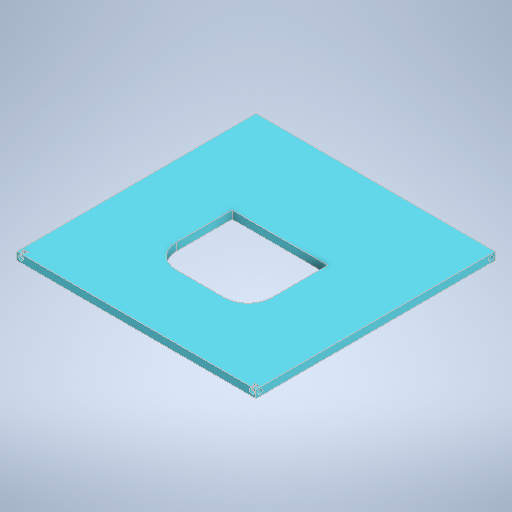
# Autodesk Inventor part: CasaJugueteAPM
Saved by Autodesk Inventor 2025.2 (Build 292293000, 293)
## iProperties
Created: 2024-11-26
Part Number: CasaJugueteAPM
Material: Plástico ABS
Document SubType Name: Modeling
Designer: usuario
Density: 1.06 g/cm^3
Appearance: Suave - Negro
Author: usuario
Autodesk Inventor part; units mm, degrees
ref_plane "YZ Plane" through (0, 0, 0) normal (1, 0, 0) x (0, 1, 0)
ref_plane "XZ Plane" through (0, 0, 0) normal (0, 1, 0) x (-1, 0, 0)
ref_plane "XY Plane" through (0, 0, 0) normal (0, 0, 1) x (1, 0, 0)
sketch "Boceto1" plane through (0, 0, 0) normal (0, 0, 1) x (1, 0, 0)
  line L0 (0, 0) -> (150, 0)
  line L1 (150, 0) -> (150, 150)
  line L2 (150, 150) -> (0, 150)
  line L3 (0, 150) -> (0, 0)
  line L4 (5, 145) -> (145, 145)
  line L5 (145, 145) -> (145, 5)
  line L6 (145, 5) -> (5, 5)
  line L7 (5, 5) -> (5, 145)
  dimension "d0" = 150
  dimension "d1" = 150
  dimension "d2" = 5
  constraints: 16 end point, 4 parallel, 2 perpendicular, 1 horizontal, 3 other
  measures "d0" distance of L2.end L1.end
  measures "d1" distance of L1.end L0.end
  measures "d2" distance between parallel lines of L2 L4
extrude "Extrusión1" add sketch "Boceto1" along normal blind 150
sketch "Boceto2" plane through (150, 0, 0) normal (1, 0, 0) x (0, 0, -1)
  line L0 (-150, 0) -> (-150, 150) projected
  line L1 (-150, 75) -> (-190, 75) construction
  line L2 (-190, 75) -> (-150, 150)
  line L3 (0, 0) -> (-150, 0) construction
  line L4 (-150, 0) -> (-190, 75)
  dimension "d5" = 40
  constraints: 6 end point, 1 horizontal, 1 midpoint
  measures "d5" distance of L1.start L1.end
extrude "Extrusión2" add sketch "Boceto2" against normal blind 5
ref_plane "Plano de trabajo1" through (75, 0, 0) normal (1, 0, 0) x (0, 0, -1)
mirror "Simetría1" about plane through (75, 0, 0) normal (1, 0, 0) of "Extrusión2"
sketch "Boceto3" plane through (0, 150, 0) normal (0, 1, 0) x (1, 0, 0)
  line L0 (105, -60) -> (45, -60)
  line L1 (45, -60) -> (45, -95)
  line L2 (60, -110) -> (90, -110)
  line L3 (105, -95) -> (105, -60)
  line L4 (150, 0) -> (0, 0) projected
  line L5 (145, -150) -> (5, -150) projected
  arc A0 (90, -110) -> (105, -95) centre (90, -95) ccw
  arc A1 (45, -95) -> (60, -110) centre (60, -95) ccw
  point P0 (45, -110)
  point P1 (105, -110)
  point P2 (75, -60)
  point P3 (75, 0)
  dimension "d8" = 60
  dimension "d9" = 50
  dimension "d10" = 40
  dimension "d11" = 15
  constraints: 8 end point, 4 point on circle, 4 point on line, 4 tangent, 2 centre point, 2 midpoint, 2 parallel, 1 equal radius, 1 horizontal, 1 perpendicular, 1 vertical alignment
  measures "d8" distance of point (105, -110) point (45, -110)
  measures "d9" distance of point (45, -110) L0.end
  measures "d10" distance between parallel lines of L5 L2
  measures "d11" radius of A0
extrude "Extrusión3" cut sketch "Boceto3" against normal through all
sketch "Boceto4" plane through (150, 0, 0) normal (1, 0, 0) x (0, 0, -1)
  line L0 (-13, 20) -> (-123, 20)
  line L1 (-128, 25) -> (-128, 75)
  line L2 (-123, 80) -> (-13, 80)
  line L3 (-8, 75) -> (-8, 25)
  line L4 (0, 0) -> (0, 150) projected
  line L5 (0, 0) -> (-150, 0) projected
  arc A0 (-123, 80) -> (-128, 75) centre (-123, 75) ccw
  arc A1 (-8, 75) -> (-13, 80) centre (-13, 75) ccw
  arc A2 (-13, 20) -> (-8, 25) centre (-13, 25) ccw
  arc A3 (-128, 25) -> (-123, 20) centre (-123, 25) ccw
  point P0 (-128, 80)
  point P1 (-128, 20)
  point P2 (-8, 80)
  dimension "d14" = 120
  dimension "d15" = 60
  dimension "d16" = 8
  dimension "d17" = 20
  dimension "d18" = 5
  constraints: 8 end point, 8 point on circle, 8 tangent, 6 point on line, 4 centre point, 3 equal radius, 2 parallel, 1 horizontal, 1 perpendicular
  measures "d14" distance of point (-128, 80) point (-8, 80)
  measures "d15" distance of point (-128, 20) point (-128, 80)
  measures "d16" distance between parallel lines of L4 L3
  measures "d17" distance between parallel lines of L0 L5
  measures "d18" radius of A0
extrude "Extrusión4" cut sketch "Boceto4" against normal up to surface (5 mm away)
sketch "Boceto5" plane through (0, 0, 0) normal (-1, 0, 0) x (0, 0, 1)
  line L0 (65, 125) -> (115, 125)
  line L1 (120, 120) -> (120, 30)
  line L2 (115, 25) -> (65, 25)
  line L3 (60, 30) -> (60, 120)
  line L4 (0, 150) -> (0, 0) projected
  arc A0 (120, 120) -> (115, 125) centre (115, 120) ccw
  arc A1 (115, 25) -> (120, 30) centre (115, 30) ccw
  arc A2 (65, 125) -> (60, 120) centre (65, 120) ccw
  arc A3 (60, 30) -> (65, 25) centre (65, 30) ccw
  point P0 (60, 150)
  point P1 (120, 25)
  point P2 (120, 125)
  point P3 (60, 25)
  point P4 (60, 75)
  point P5 (0, 75)
  dimension "d21" = 60
  dimension "d22" = 100
  dimension "d23" = 60
  dimension "d24" = 5
  constraints: 8 end point, 8 point on circle, 8 tangent, 6 point on line, 4 centre point, 3 equal radius, 2 midpoint, 2 parallel, 1 horizontal, 1 horizontal alignment, 1 perpendicular
  measures "d21" distance of point (120, 25) point (60, 25)
  measures "d22" distance of point (120, 125) point (120, 25)
  measures "d23" distance between parallel lines of L4 L3
  measures "d24" radius of A0
extrude "Extrusión5" cut sketch "Boceto5" against normal blind 10
sketch "Boceto6" plane through (150, 0, 0) normal (1, 0, 0) x (0, 0, -1)
  line L0 (-190, 75) -> (-150, 0) projected
  line L1 (-150, 150) -> (-190, 75) projected
  line L2 (-154.4118, 152.3529) -> (-195.6667, 75)
  line L3 (-195.6667, 75) -> (-154.4118, -2.3529)
  line L4 (-154.4118, 152.3529) -> (-144.4118, 152.3529)
  line L5 (-144.4118, 152.3529) -> (-144.4118, 150)
  line L6 (-154.4118, -2.3529) -> (-144.4118, -2.3529)
  line L7 (-144.4118, -2.3529) -> (-144.4118, 0)
  line L8 (0, 0) -> (-150, 0) projected
  line L9 (0, 150) -> (-150, 150) projected
  dimension "d27" = 5
  dimension "d28" = 10
  constraints: 12 end point, 2 horizontal, 2 perpendicular, 1 other
  measures "d27" distance between parallel lines of L1 L2
  measures "d28" distance of L2.start L4.end
extrude "Extrusión6" add sketch "Boceto6" along normal blind 10 and the other way blind 160
fillet "Empalme1" radius 5 3 edges at (75, 152.3529, 154.4118) (75, 75, 195.6667) (75, -2.3529, 154.4118)
sketch "Boceto7" plane through (150, 25, 8) normal (0, 0, 1) x (1, 0, 0)
  circle A0 centre (-2.5, 2.5) radius 1.25
  line L0 (0, 50) -> (0, 0) projected
  line L1 (0, 0) -> (-5, 0) projected
  point P0 (-150, -25)
  point P1 (-2.5, 0)
  dimension "d34" = 2.5
  dimension "d35" = 2.5
  dimension "d36" = 2.5
  constraints: 1 centre point, 1 midpoint
  measures "d34" diameter of A0
  measures "d35" distance from line of L0 A0.centre
  measures "d36" distance of A0.centre point (-2.5, 0)
extrude "Extrusión7" cut sketch "Boceto7" against normal blind 3
ref_plane "Plano de trabajo2" through (150, 25, 68) normal (0, 0, 1) x (1, 0, 0)
mirror "Simetría2" about plane through (150, 25, 68) normal (0, 0, 1) of "Extrusión7"
sketch "Boceto8" plane through (160, 0, 0) normal (1, 0, 0) x (0, 0, -1)
  arc A0 (-155.8235, 0.2941) -> (-151.4118, -2.3529) centre (-151.4118, 2.6471) ccw projected
  line L0 (-151.4118, -2.3529) -> (-144.4118, -2.3529) projected
  line L1 (-144.4118, -2.3529) -> (-144.4118, 0) projected
  line L2 (-144.4118, 0) -> (-150, 0) projected
  line L3 (-150, 0) -> (-190, 75) projected
  line L4 (-190, 75) -> (-150, 150) projected
  line L5 (-150, 150) -> (-144.4118, 150) projected
  line L6 (-144.4118, 150) -> (-144.4118, 152.3529) projected
  line L7 (-144.4118, 152.3529) -> (-151.4118, 152.3529) projected
  arc A1 (-151.4118, 152.3529) -> (-155.8235, 149.7059) centre (-151.4118, 147.3529) ccw projected
  line L8 (-155.8235, 149.7059) -> (-194.4118, 77.3529) projected
  arc A2 (-194.4118, 77.3529) -> (-194.4118, 72.6471) centre (-190, 75) ccw projected
  line L9 (-194.4118, 72.6471) -> (-155.8235, 0.2941) projected
  point P0 (0, 0)
extrude "Extrusión8" cut sketch "Boceto8" against normal through all
sketch "Boceto9" plane through (145, 0, 150) normal (0, -0.4705882, 0.8823529) x (1, 0, 0)
  circle A0 centre (2.5, 2.5) radius 1.5
  line L0 (5, 85) -> (5, 0) projected
  line L1 (5, 0) -> (0, 0) projected
  point P0 (-145, -70.5882)
  dimension "d41" = 3
  dimension "d42" = 2.5
  dimension "d43" = 2.5
  constraints: 1 centre point
  measures "d41" diameter of A0
  measures "d42" distance from line of L0 A0.centre
  measures "d43" distance from line of L1 A0.centre
extrude "Extrusión9" cut sketch "Boceto9" against normal blind 5
ref_plane "Plano de trabajo3" through (75, 0, 0) normal (1, 0, 0) x (0, 0, -1)
ref_plane "Plano de trabajo4" through (0, 75, 0) normal (0, -1, 0) x (1, 0, 0)
mirror "Simetría3" about plane through (75, 0, 0) normal (1, 0, 0) of "Extrusión9"
mirror "Simetría4" about plane through (0, 75, 0) normal (0, -1, 0) of "Extrusión8", "Extrusión9", "Simetría3"
sketch "Boceto10" plane through (0, 150, 0) normal (0, 1, 0) x (1, 0, 0)
  line L0 (5, -115) -> (5, -65) projected
  arc A0 (45, -95) -> (60, -110) centre (60, -95) ccw projected
  line L1 (45, -95) -> (45, -60) projected
  line L2 (45, -60) -> (105, -60) projected
  line L3 (105, -60) -> (105, -95) projected
  arc A1 (90, -110) -> (105, -95) centre (90, -95) ccw projected
  line L4 (90, -110) -> (60, -110) projected
  line L5 (150, 0) -> (150, -150) projected
  line L6 (150, 0) -> (0, 0) projected
  line L7 (0, 0) -> (0, -150) projected
  line L8 (5, -150) -> (0, -150) projected
  line L9 (145, -150) -> (5, -150) projected
  line L10 (150, -150) -> (145, -150) projected
extrude "Extrusión10" cut sketch "Boceto10" against normal up to surface (145 mm away)
sketch "Boceto11" plane through (150, 0, 150) normal (1, 0, 0) x (0, 0, -1)
  line L0 (0, 0) -> (0, 5) projected
  line L1 (0, 5) -> (0, 150) projected
  line L2 (-40, 75) -> (0, 0) projected
  line L3 (0, 150) -> (-40, 75) projected
  point P0 (150, 0)
extrude "Extrusión11" cut sketch "Boceto11" against normal through all
sketch "Boceto12" plane through (150, 0, 0) normal (1, 0, 0) x (0, 0, -1)
  circle A0 centre (-147.5, 2.5) radius 1.5
  line L0 (0, 5) -> (-150, 5) projected
  line L1 (-150, 5) -> (-150, 0) projected
  line L2 (-75, 5) -> (-75, -25.1445) construction
  circle A1 centre (-2.5, 2.5) radius 1.5
  point P0 (0, 0)
  dimension "d50" = 3
  dimension "d51" = 2.5
  dimension "d52" = 2.5
  constraints: 2 centre point, 2 end point, 1 midpoint, 1 symmetric about line, 1 vertical, 1 other
  measures "d50" diameter of A0
  measures "d51" distance from line of L0 A0.centre
  measures "d52" distance from line of L1 A0.centre
extrude "Extrusión12" cut sketch "Boceto12" against normal blind 5
mirror "Simetría5" about plane through (75, 0, 0) normal (1, 0, 0) of "Extrusión12"
